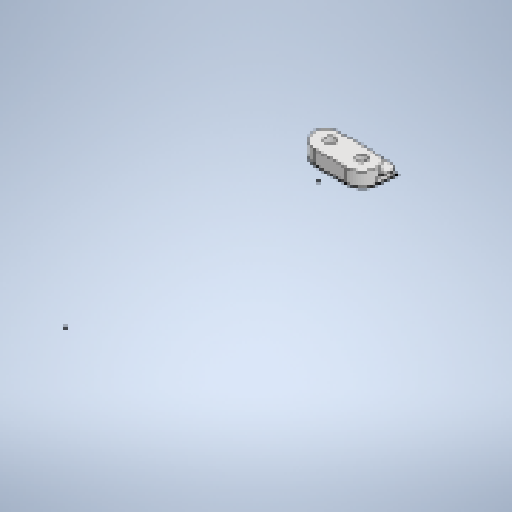
# Autodesk Inventor part: Thrust Bushing
Saved by Autodesk Inventor 2023.4 (Build 274418000, 418)
## iProperties
Created: 2024-04-30
Part Number: Thrust Bushing
Material: UHMW, White
Document SubType Name: Modeling
Designer: Nathan Cai
Density: 0.94 g/cm^3
Appearance: Smooth - White
Mass: 0.58909 g
Surface Area: 6.52842 cm^2
Volume: 0.626692 cm^3
Author: Nathan Cai
Autodesk Inventor part; units mm, degrees
ref_plane "YZ Plane" through (0, 0, 0) normal (1, 0, 0) x (0, 1, 0)
ref_plane "XZ Plane" through (0, 0, 0) normal (0, 1, 0) x (-1, 0, 0)
ref_plane "XY Plane" through (0, 0, 0) normal (0, 0, 1) x (1, 0, 0)
sketch "Sketch1" plane through (0, 0, 0) normal (0, 1, 0) x (-1, 0, 0)
  circle A0 centre (0, 0) radius 4.7625 construction
  line L0 (4.7625, 0) -> (-4.7625, 0) construction
  circle A1 centre (4.7625, 0) radius 1.5
  circle A2 centre (4.7625, 0) radius 3.5
  circle A3 centre (-4.7625, 0) radius 1.5
  circle A4 centre (-4.7625, 0) radius 3.5
  line L1 (0, 0) -> (0, 4.7625) construction
  arc A5 (-4.9577, -3.4946) -> (4.9577, -3.4946) centre (0, 85.2671) ccw construction
  arc A6 (-9.8858, -2.9537) -> (9.8858, -2.9537) centre (0, 85.2671) ccw
  arc A7 (-10.1651, -5.4464) -> (10.1651, -5.4464) centre (0, 85.2671) ccw
  arc A8 (7.1041, -4.1471) -> (1.5249, -3.4928) centre (4.7625, 0) ccw
  arc A9 (-1.5249, -3.4928) -> (-7.1041, -4.1471) centre (-4.7625, 0) ccw
  arc A10 (-7.1041, -4.1471) -> (7.1041, -4.1471) centre (0, 8.4348) ccw
  line L2 (4.7625, 4.7625) -> (-4.7625, 4.7625)
  line L3 (10.1651, -5.4464) -> (9.4954, 0.5304)
  line L4 (-9.4954, 0.5304) -> (-10.1651, -5.4464)
  point P0 (-8.3689, -3.1105)
  point P1 (8.3689, -3.1105)
  point P2 (0, -6.0141)
  dimension "d2" = 7
  dimension "d4" = 7
  dimension "d0" = 9.525
  dimension "d1" = 3
  dimension "d3" = 3
  dimension "d5" = 88.9
  dimension "d6" = 0.127
  dimension "d7" = 2.3813
  dimension "d8" = 9.525
  dimension "d9" = 9.525
  constraints: 25 point on circle, 10 end point, 9 centre point, 7 coincident, 6 tangent, 2 horizontal, 2 line through centre, 2 point on line, 1 midpoint, 1 vertical, 8 other
  measures "d0" diameter of A0
  measures "d1" diameter of A1
  measures "d3" diameter of A3
  measures "d5" radius of A5
  measures "d6" radial gap between concentric circles of A5 A6
  measures "d7" radial gap between concentric circles of A5 A7
  measures "d8" diameter of A8
  measures "d9" diameter of A9
extrude "Extrusion1" add sketch "Sketch1" along normal blind 1.625
extrude "Extrusion2" add sketch "Sketch1" along normal blind 4.25 contours A2 A6 | A2 A6 A8 | A6 A9 A8 | A6 A4 A9 | A9 L2 A8 | A6 A4 picked at (7.5452, 0.4078) picked at (-1.9781, 0.4008)
fillet "Fillet1" radius 3.175 2 edges at (8.3689, 2.9375, -3.1105) (-8.3689, 2.9375, -3.1105)
fillet "Fillet2" radius 1.5875 2 edges at (-10.1651, 0.8125, -5.4464) (10.1651, 0.8125, -5.4464)
chamfer "Chamfer1" distance 0.1 angle 45 5 edges at (0, 1.625, -6.0141) (-9.6409, 1.625, -5.0331) (-9.7411, 1.625, -1.6622) (9.6409, 1.625, -5.0331) (9.7411, 1.625, -1.6622)
body "Solid1"
